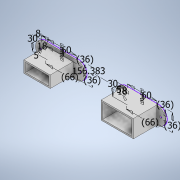
# Autodesk Inventor part: single_chamber_EIT_test
Saved by Autodesk Inventor 2021 (Build 250183000, 183)
## iProperties
Created: 2021-04-07
Part Number: single_chamber_EIT_test
Material: Generic
Document SubType Name: Modeling
Designer: Charlie
Density: 1 g/cm^3
Appearance: Default
Author: Charlie
Autodesk Inventor part; units mm, degrees
ref_plane "YZ Plane" through (0, 0, 0) normal (1, 0, 0) x (0, 1, 0)
ref_plane "XZ Plane" through (0, 0, 0) normal (0, 1, 0) x (-1, 0, 0)
ref_plane "XY Plane" through (0, 0, 0) normal (0, 0, 1) x (1, 0, 0)
sketch "outer mould sketch" plane through (0, 0, 0) normal (0, 0, 1) x (1, 0, 0)
  line L0 (30, 15) -> (-30, 15)
  line L1 (-30, 15) -> (-30, -15)
  line L2 (-30, -15) -> (30, -15)
  line L3 (30, -15) -> (30, 15)
  line L4 (-27, 12) -> (27, 12)
  line L5 (27, 12) -> (27, -12)
  line L6 (27, -12) -> (-27, -12)
  line L7 (-27, -12) -> (-27, 12)
  line L8 (-33, 18) -> (33, 18)
  line L9 (33, 18) -> (33, -18)
  line L10 (33, -18) -> (-33, -18)
  line L11 (-33, -18) -> (-33, 18)
  arc A0 (-33, 18) -> (-33, -18) centre (-33, 0) ccw
  circle A1 centre (-41, 0) radius 2.5
  line L12 (0, -18) -> (0, 18) construction
  arc A2 (33, -18) -> (33, 18) centre (33, 0) ccw
  circle A3 centre (41, 0) radius 2.5
  dimension "d15" = 30
  dimension "d16" = 60
  dimension "d17" = 3
  dimension "d18" = 3
  dimension "d19" = 18
  dimension "d20" = 5
  dimension "d21" = 8
  dimension "d22" = 36
  dimension "d24" = 66
  dimension "d25" = 36
  constraints: 26 end point, 6 parallel, 4 centre point, 4 point on circle, 3 perpendicular, 2 midpoint, 2 symmetric about line, 8 other
  measures "d15" distance of L0.end L1.end
  measures "d16" distance of L0.start L0.end
  measures "d17" distance between parallel lines of L0 L4
  measures "d18" distance between parallel lines of L0 L8
  measures "d19" radius of A0
  measures "d20" diameter of A1
  measures "d21" distance from line of L11 A1.centre
  measures "d22" distance between parallel lines of L10 L8
  measures "d24" distance of L9.end L10.end
  measures "d25" distance of L8.end L9.end
extrude "Extrusion1" add sketch "outer mould sketch" along normal blind 3 contours L11 A0 | A2 L9
extrude "Extrusion2" add sketch "outer mould sketch" along normal blind 51 contours L8 L9 L10 L11
sketch "Sketch5" plane through (0, 0, 0) normal (0, 0, 1) x (1, 0, 0)
  line L0 (-134.3835, 13.0664) -> (-194.3835, 13.0664)
  line L1 (-194.3835, 13.0664) -> (-194.3835, -16.9336)
  line L2 (-194.3835, -16.9336) -> (-134.3835, -16.9336)
  line L3 (-134.3835, -16.9336) -> (-134.3835, 13.0664)
  line L4 (-191.3835, 10.0664) -> (-137.3835, 10.0664)
  line L5 (-137.3835, 10.0664) -> (-137.3835, -13.9336)
  line L6 (-137.3835, -13.9336) -> (-191.3835, -13.9336)
  line L7 (-191.3835, -13.9336) -> (-191.3835, 10.0664)
  line L8 (-197.3835, 16.0664) -> (-131.3835, 16.0664)
  line L9 (-131.3835, 16.0664) -> (-131.3835, -19.9336)
  line L10 (-131.3835, -19.9336) -> (-197.3835, -19.9336)
  line L11 (-197.3835, -19.9336) -> (-197.3835, 16.0664)
  arc A0 (-197.3835, 16.0664) -> (-197.3835, -19.9336) centre (-197.3835, -1.9336) ccw
  circle A1 centre (-41.0005, 0) radius 2.5
  line L12 (-164.3835, -19.9336) -> (-164.3835, 16.0664) construction
  arc A2 (-131.3835, -19.9336) -> (-131.3835, 16.0664) centre (-131.3835, -1.9336) ccw
  circle A3 centre (41, 0) radius 2.5
  line L13 (-197.3835, -1.9336) -> (-215.3835, -1.9336) construction
  circle A4 centre (-205.3835, -1.9336) radius 2.5
  circle A5 centre (-123.3835, -1.9336) radius 2.5
  line L14 (-140.3835, 7.0664) -> (-188.3835, 7.0664)
  line L15 (-188.3835, 7.0664) -> (-188.3835, -10.9336)
  line L16 (-188.3835, -10.9336) -> (-140.3835, -10.9336)
  line L17 (-140.3835, -10.9336) -> (-140.3835, 7.0664)
  point P0 (0, 0)
  dimension "d26" = 30
  dimension "d27" = 60
  dimension "d28" = 3
  dimension "d29" = 3
  dimension "d30" = 18
  dimension "d31" = 5
  dimension "d32" = 156.383
  dimension "d33" = 36
  dimension "d34" = 66
  dimension "d35" = 36
  dimension "d36" = 5
  dimension "d37" = 8
  dimension "d42" = 3
  constraints: 36 end point, 8 parallel, 6 centre point, 5 point on circle, 4 perpendicular, 2 midpoint, 2 symmetric about line, 1 point on line, 11 other
  measures "d26" distance of L1.start L1.end
  measures "d27" distance of L0.start L1.start
  measures "d28" distance between parallel lines of L0 L4
  measures "d29" distance between parallel lines of L0 L8
  measures "d30" radius of A0
  measures "d31" diameter of A1
  measures "d32" distance from line of L11 A1.centre
  measures "d33" distance between parallel lines of L10 L8
  measures "d34" distance of L10.start L11.start
  measures "d35" distance of L8.end L10.start
  measures "d36" diameter of A4
  measures "d37" distance from line of L11 A4.centre
  measures "d42" distance between parallel lines of L4 L14
extrude "Extrusion5" add sketch "Sketch5" along normal blind 51 separate body contours L4 L5 L6 L7
extrude "Extrusion4" add sketch "Sketch5" along normal blind 3 contours L3 L2 L1 L0 | L4 L5 L6 L7 | L8 L9 L10 L11 | L11 A0 | A2 L9 | L17 L16 L15 L14 bodies 2
body "Solid1"
body "Solid2"
